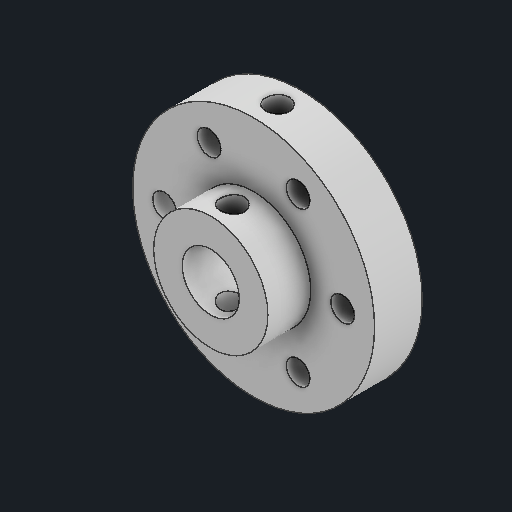
# Autodesk Inventor part: PololuHub1994
Saved by Autodesk Inventor 2025.2 (Build 292293000, 293)
## iProperties
Created: 2025-09-15
Part Number: PololuHub1994
Material: Generic
Document SubType Name: Modeling
Designer: valer
Density: 1 g/cm^3
Appearance: Default
Author: valer
Autodesk Inventor part; units mm, degrees
ref_plane "YZ Plane" through (0, 0, 0) normal (1, 0, 0) x (0, 1, 0)
ref_plane "XZ Plane" through (0, 0, 0) normal (0, 1, 0) x (-1, 0, 0)
ref_plane "XY Plane" through (0, 0, 0) normal (0, 0, 1) x (1, 0, 0)
sketch "Base" plane through (0, 0, 0) normal (0, 0, 1) x (1, 0, 0)
  circle A0 centre (0, 0) radius 3
  circle A1 centre (0, 0) radius 6
  circle A2 centre (0, 0) radius 12.7
  circle A3 centre (0, 0) radius 9.35 construction
  line L0 (0, 6) -> (0, 12.7) construction
  line L1 (0, -17.78) -> (0, 17.78) construction
  circle A4 centre (-9.35, 0) radius 1.25
  line L2 (-17.78, 0) -> (17.78, 0) construction
  circle A5 centre (-4.675, -8.0973) radius 1.25
  circle A6 centre (4.675, -8.0973) radius 1.25
  circle A7 centre (9.35, 0) radius 1.25
  circle A8 centre (4.675, 8.0973) radius 1.25
  circle A9 centre (-4.675, 8.0973) radius 1.25
  point P0 (0, 9.35)
  dimension "d1" = 12
  dimension "d2" = 25.4
  dimension "d0" = 6
  dimension "d3" = 2.5
  dimension "d6" = 360
  constraints: 8 centre point, 4 coincident, 2 end point, 2 point on circle, 2 vertical alignment, 1 collinear, 1 midpoint, 1 point on line, 1 vertical, 17 other
  measures "d0" diameter of A0
  measures "d3" diameter of A4
extrude "BaseFeature" add sketch "Base" against normal blind 5 contours A1 | A2
extrude "FlangeFeature" add sketch "Base" along normal blind 4.5 contours A1
sketch "FixatingHoles" plane through (0, 0, 0) normal (0, 1, 0) x (-1, 0, 0)
  line L0 (-3, 4.5) -> (3, 4.5) construction
  line L1 (0, 4.5) -> (0, 0) construction
  line L2 (12.7, 0) -> (-12.7, 0) projected
  line L3 (3, -5) -> (-3, -5) construction
  line L4 (0, -5) -> (0, 0) construction
  circle A0 centre (0, 2.25) radius 1.25
  circle A1 centre (0, -2.5) radius 1.25
  dimension "d12" = 2.5
  dimension "d13" = 2.5
  constraints: 4 end point, 4 midpoint, 2 centre point, 1 collinear, 1 perpendicular
  measures "d12" diameter of A0
  measures "d13" diameter of A1
extrude "FixatingHolesFeature" cut sketch "FixatingHoles" along normal through all both and the other way through all
body "Solid1"
